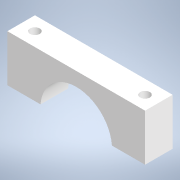
# Autodesk Inventor part: motortarto
Saved by Autodesk Inventor 2022 (Build 260153000, 153)
## iProperties
Created: 2021-10-06
Part Number: motortarto
Material: ABS Plastic
Document SubType Name: Modeling
Designer: Varga Tamás
Density: 1.06 g/cm^3
Appearance: Smooth - White
Mass: 6.12466 g
Surface Area: 30.2554 cm^2
Volume: 5.77798 cm^3
Author: Varga Tamás
Autodesk Inventor part; units mm, degrees
ref_plane "YZ Plane" through (0, 0, 0) normal (1, 0, 0) x (0, 1, 0)
ref_plane "XZ Plane" through (0, 0, 0) normal (0, 1, 0) x (-1, 0, 0)
ref_plane "XY Plane" through (0, 0, 0) normal (0, 0, 1) x (1, 0, 0)
sketch "Sketch1" plane through (0, 0, 0) normal (0, 0, 1) x (1, 0, 0)
  line L0 (0, 0) -> (30, 0)
  line L1 (30, 0) -> (30, 35)
  line L2 (30, 35) -> (0, 35)
  line L3 (0, 35) -> (0, 0)
  circle A0 centre (15, 17) radius 13
  dimension "d0" = 30
  dimension "d1" = 35
  dimension "d2" = 26
  dimension "d3" = 15
  dimension "d4" = 18
  constraints: 8 end point, 2 parallel, 1 centre point, 1 horizontal, 1 perpendicular
  measures "d0" distance of L2.end L1.end
  measures "d1" distance of L0.end L1.end
  measures "d2" diameter of A0
  measures "d3" distance from line of L1 A0.centre
  measures "d4" distance from line of L2 A0.centre
extrude "Extrusion1" add sketch "Sketch1" along normal blind 10
sketch "Sketch4" plane through (30, 0, 0) normal (1, 0, 0) x (0, 0, -1)
  line L0 (0, 0) -> (-10, 0) projected
  line L1 (0, 0) -> (0, 35) projected
  line L2 (-10, 0) -> (0, 0)
  line L3 (0, 0) -> (0, 18)
  line L4 (0, 18) -> (-10, 18)
  line L5 (-10, 18) -> (-10, 0)
  dimension "d25" = 18
  constraints: 8 end point, 2 parallel, 1 horizontal, 1 perpendicular, 1 point on line
  measures "d25" distance between parallel lines of L4 L0
extrude "Extrusion2" cut sketch "Sketch4" against normal through all
sketch "Sketch5" plane through (30, 35, 10) normal (1, 0, 0) x (0, 0, -1)
  line L0 (10, 0) -> (10, -17) projected
  line L1 (0, 0) -> (0, -17) projected
  line L2 (10, -17) -> (0, -17)
  line L3 (0, -17) -> (0, 0)
  line L4 (0, 0) -> (10, 0)
  line L5 (10, 0) -> (10, -17)
  point P0 (10, -35)
  constraints: 8 end point, 2 parallel, 1 horizontal, 1 perpendicular
extrude "Extrusion3" add sketch "Sketch5" along normal blind 10
sketch "Sketch6" plane through (0, 35, 0) normal (-1, 0, 0) x (0, 0, 1)
  line L0 (0, -17) -> (0, 0) projected
  line L1 (10, -17) -> (0, -17)
  line L2 (0, -17) -> (0, 0)
  line L3 (0, 0) -> (10, 0)
  line L4 (10, 0) -> (10, -17)
  point P0 (0, -35)
  constraints: 8 end point, 2 parallel, 1 horizontal, 1 perpendicular
extrude "Extrusion4" add sketch "Sketch6" along normal blind 10
sketch "Sketch7" plane through (40, 35, 10) normal (0, 1, 0) x (1, 0, 0)
  circle A0 centre (-45, 5) radius 1.75
  circle A1 centre (-5, 5) radius 1.75
  line L0 (-50, 0) -> (-50, 10) projected
  line L1 (-50, 10) -> (0, 10) projected
  line L2 (0, 10) -> (0, 0) projected
  point P0 (-40, 10)
  dimension "d32" = 3.5
  dimension "d33" = 3.5
  dimension "d34" = 5
  dimension "d35" = 5
  dimension "d36" = 5
  dimension "d37" = 5
  constraints: 2 centre point
  measures "d32" diameter of A0
  measures "d33" diameter of A1
  measures "d34" distance from line of L0 A0.centre
  measures "d35" distance from line of L1 A0.centre
  measures "d36" distance from line of L1 A1.centre
  measures "d37" distance from line of L2 A1.centre
extrude "Extrusion5" cut sketch "Sketch7" against normal through all
body "Solid1"
